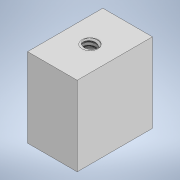
# Autodesk Inventor part: Part1
Saved by Autodesk Inventor 2020.3 (Build 243373000, 373)
## iProperties
Created: 2020-05-27
Part Number: Part1
Material: Generic
Document SubType Name: Modeling
Designer: robst
Density: 1 g/cm^3
Appearance: Default
Author: robst
Autodesk Inventor part; units mm, degrees
ref_plane "YZ Plane" through (0, 0, 0) normal (1, 0, 0) x (0, 1, 0)
ref_plane "XZ Plane" through (0, 0, 0) normal (0, 1, 0) x (-1, 0, 0)
ref_plane "XY Plane" through (0, 0, 0) normal (0, 0, 1) x (1, 0, 0)
sketch "Sketch1" plane through (0, 0, 0) normal (0, 1, 0) x (-1, 0, 0)
  line L0 (-7.9423, 12.0459) -> (-7.9423, -12.0459)
  line L1 (-7.9423, -12.0459) -> (7.9423, -12.0459)
  line L2 (7.9423, -12.0459) -> (7.9423, 12.0459)
  line L3 (7.9423, 12.0459) -> (-7.9423, 12.0459)
  line L4 (-7.9423, 12.0459) -> (7.9423, -12.0459) construction
  line L5 (-7.9423, -12.0459) -> (7.9423, 12.0459) construction
  point P0 (0, 0)
  constraints: 12 end point, 2 midpoint, 2 parallel, 1 perpendicular, 1 vertical
extrude "Extrusion1" add sketch "Sketch1" against normal blind 25.4
sketch "Sketch2" plane through (0, 0, 0) normal (0, 1, 0) x (1, 0, 0)
  circle A0 centre (0, 0) radius 2.5527
  dimension "d2" = 5.1054
  constraints: 1 centre point, 1 coincident
  measures "d2" diameter of A0
extrude "Extrusion2" cut sketch "Sketch2" against normal blind 25.4
thread "Thread1" size "1/4-20 UNC" class "2B" standard "ANSI Unified Screw Threads" full length
sketch "Sketch4" plane through (0, -25.4, 0) normal (-1, 0, 0) x (0, 0, 1)
  line L0 (2.5527, 0) -> (2.5527, 25.4)
  line L1 (2.5527, 25.4) -> (1.8653, 25.4)
  line L2 (1.8653, 25.4) -> (1.8653, 0)
  line L3 (1.8653, 0) -> (2.5527, 0)
  line L4 (0, -6.6992) -> (0, 30.7499) projected
  constraints: 8 end point
revolve "Revolution1" add sketch "Sketch4" angle 360 about axis through (0, -25.4, 0) along (0, 1, 0) separate body
sketch "Sketch3" plane through (0, -25.4, 2.5527) normal (1, 0, 0) x (0, 1, 0)
  line L0 (-0.635, 0.275) -> (-0.8396, -0.0794) construction
  line L1 (-0.635, 0.275) -> (-0.4304, -0.0794) construction
  line L2 (-0.635, 0.275) -> (-0.635, 0) construction
  line L3 (-0.7938, 0) -> (-0.7021, 0) construction
  line L4 (0, -0.8249) -> (0.0794, -0.6874) construction
  line L5 (-1.27, -0.8249) -> (-1.3494, -0.6874) construction
  line L6 (-1.3494, -0.6874) -> (-1.27, -0.6874) construction
  line L7 (-1.1906, -0.6874) -> (-1.27, -0.8249) construction
  arc A0 (-0.7021, 0) -> (-0.8396, -0.0794) centre (-0.7021, -0.1587) ccw
  arc A1 (-0.4304, -0.0794) -> (-0.5679, 0) centre (-0.5679, -0.1587) ccw
  line L8 (0, -0.8249) -> (0, -0.6874) construction
  line L9 (-1.27, -0.8249) -> (-1.27, -0.6874) construction
  arc A2 (-0.1023, -0.6477) -> (-0.0335, -0.6874) centre (-0.0335, -0.608) ccw
  line L10 (-0.4304, -0.0794) -> (-0.1023, -0.6477)
  line L11 (-0.7021, 0) -> (-0.5679, 0)
  line L12 (-0.8396, -0.0794) -> (-1.1677, -0.6477)
  line L13 (-0.0335, -0.6874) -> (0, -0.6874) construction
  line L14 (0, -0.6874) -> (0.0794, -0.6874) construction
  arc A3 (-1.2365, -0.6874) -> (-1.1677, -0.6477) centre (-1.2365, -0.608) ccw
  line L15 (-1.1677, -0.6477) -> (-1.1906, -0.6874) construction
  line L16 (-1.27, -0.6874) -> (-1.2365, -0.6874) construction
  line L17 (-1.2365, -0.6874) -> (-0.0335, -0.6874)
  line L18 (0, 0) -> (0.4413, 0)
  line L19 (0, 0) -> (0, 0.419)
  line L20 (0, -0.8249) -> (-0.1023, -0.6477) construction
  dimension "d7" = 0.275
  dimension "d8" = 0.1588
  dimension "d9" = 0.0794
  dimension "d10" = 0.1375
  dimension "d11" = 1.27
  dimension "Sketch3_MajorRadius" = 0.6874
  dimension "d13" = 60
  dimension "Sketch3_ThreadOffset" = 0
  dimension "Sketch3_MinorRadius" = 0
  constraints: 42 end point, 17 tangent, 8 point on circle, 6 parallel, 5 collinear, 4 centre point, 3 point on line, 3 vertical, 2 equal radius, 2 horizontal, 2 perpendicular, 1 equal length, 1 midpoint, 4 other
  measures "d7" distance from line of L0.start L3
  measures "d8" radius of A0
  measures "d9" radius of A2
  measures "d10" distance from line of L14 L4.start
  measures "d11" distance between parallel lines of L8 L9
  measures "Sketch3_MajorRadius" distance between parallel lines of L14 L18
  measures "d13" angle of L10 L12
  measures "Sketch3_ThreadOffset" distance between parallel lines of L19 L8
  measures "Sketch3_MinorRadius" distance between parallel lines of L18 L11
coil "Coil1" sketch "Sketch3" operation cut axis through (0, -25.4, 0) along (0, 1, 0) pitch 1.2713 turns 21.978022 hand right bodies 2
equation "\"d7\" = 0.216506 * Sketch3_Pitch"
equation "\"d8\" = d16"
equation "\"d9\" = 0.0625 * Sketch3_Pitch"
equation "\"d10\" = 0.108253 * Sketch3_Pitch"
equation "\"d11\" = Sketch3_Pitch"
equation "\"d13\" = d18"
equation "\"d16\" = 0.125 * Sketch3_Pitch"
equation "\"Sketch3_Pitch\" = 1.27"
equation "\"d18\" = 60deg"
body "Solid1"
body "Solid2"
